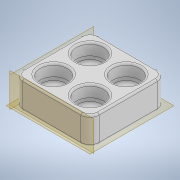
# Autodesk Inventor part: Test_Well2x2
Saved by Autodesk Inventor 2022 (Build 260153000, 153)
## iProperties
Created: 2021-11-23
Part Number: Test_Well2x2
Material: Generic
Document SubType Name: Modeling
Designer: Gareth
Density: 1 g/cm^3
Appearance: Default
Author: Gareth
Autodesk Inventor part; units mm, degrees
sketch "Sketch1" plane through (0, 0, 0) normal (0, 1, 0) x (-1, 0, 0)
  line L0 (0, 0) -> (-42, 0)
  line L1 (-42, 0) -> (-42, -42)
  line L2 (-42, -42) -> (0, -42)
  line L3 (0, -42) -> (0, 0)
  dimension "d0" = 42
  dimension "d1" = 42
  constraints: 8 end point, 2 parallel, 1 horizontal, 1 perpendicular
  measures "d0" distance of L1.end L2.end
  measures "d1" distance of L0.end L1.end
extrude "Extrusion1" add sketch "Sketch1" along normal blind 15
sketch "Sketch2" plane through (0, 15, 0) normal (0, 1, 0) x (1, 0, 0)
  line L0 (42, 42) -> (0, 42) projected
  line L1 (0, 42) -> (0, 0) projected
  line L2 (42, 0) -> (42, 42) projected
  line L3 (0, 0) -> (42, 0) projected
  circle A0 centre (11, 31) radius 7.5
  dimension "d4" = 15
  dimension "d5" = 11
  dimension "d6" = 11
  constraints: 1 centre point
  measures "d4" diameter of A0
  measures "d5" distance from line of L0 A0.centre
  measures "d6" distance from line of L1 A0.centre
extrude "Extrusion2" cut sketch "Sketch2" against normal blind 7.5 contours A0
fillet "Fillet1" radius 1 2 edges at (3.5, 7.5, -31) (3.5, 15, -31)
pattern_linear "Rectangular Pattern2" count 2 spacing 20 along (1, 0, 0) of "Extrusion2", "Fillet1"
pattern_linear "Rectangular Pattern3" count 2 spacing 20 along (0, 0, 1) of "Extrusion2", "Fillet1", "Rectangular Pattern2"
fillet "Fillet2" radius 5 4 edges at (0, 7.5, 0) (42, 7.5, 0) (0, 7.5, -42) (42, 7.5, -42)
fillet "Fillet3" radius 1 16 edges at (21, 15, -42) (1.4645, 15, -40.5355) (0, 15, -21) (1.4645, 15, -1.4645) (21, 15, 0) (40.5355, 15, -1.4645) (42, 15, -21) (40.5355, 15, -40.5355) (1.4645, 0, -40.5355) (0, 0, -21) (1.4645, 0, -1.4645) (21, 0, 0) (40.5355, 0, -1.4645) (42, 0, -21) (40.5355, 0, -40.5355) (21, 0, -42)
body "Solid1"
